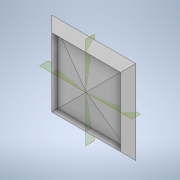
# Autodesk Inventor part: clear-square-inset
Saved by Autodesk Inventor 2021 (Build 250183000, 183)
## iProperties
Created: 2020-12-08
Part Number: clear-square-inset
Material: Generic
Document SubType Name: Modeling
Designer: Luke Kamols
Density: 1 g/cm^3
Appearance: Default
Author: Luke Kamols
Autodesk Inventor part; units mm, degrees
ref_plane "YZ Plane" through (0, 0, 0) normal (1, 0, 0) x (0, 1, 0)
ref_plane "XZ Plane" through (0, 0, 0) normal (0, 1, 0) x (-1, 0, 0)
ref_plane "XY Plane" through (0, 0, 0) normal (0, 0, 1) x (1, 0, 0)
sketch "Sketch1" plane through (0, 0, 0) normal (0, 0, 1) x (1, 0, 0)
  line L0 (0, 0) -> (44, 0)
  line L1 (44, 0) -> (44, 44)
  line L2 (44, 44) -> (0, 44)
  line L3 (0, 44) -> (0, 0)
  dimension "d0" = 44
  dimension "d1" = 44
  constraints: 8 end point, 2 parallel, 1 horizontal, 1 perpendicular
  measures "d0" distance of L2.end L1.end
  measures "d1" distance of L1.end L0.end
extrude "Extrusion1" add sketch "Sketch1" along normal blind 4
chamfer "Chamfer1" distance 4 angle 45 4 edges at (22, 44, 4) (44, 22, 4) (22, 0, 4) (0, 22, 4)
ref_plane "Work Plane1" through (0, 22, 22) normal (0, -1, 0) x (1, 0, 0)
sketch "Sketch5" plane through (0, 22, 22) normal (0, -1, 0) x (1, 0, 0)
  line L0 (40, -18) -> (4, -18) projected
  line L1 (4, -18) -> (0, -22) projected
  line L2 (0, -22) -> (44, -22) projected
  line L3 (40, -18) -> (44, -22) projected
  line L4 (4, -18) -> (4, -22)
  line L5 (40, -18) -> (40, -22)
  line L6 (40, -22) -> (40, -21)
  line L7 (40, -21) -> (22, -18)
  line L8 (4, -22) -> (4, -21)
  line L9 (22, -18) -> (4, -21)
  dimension "d25" = 1
  constraints: 12 end point, 4 point on line, 2 vertical, 1 midpoint
  measures "d25" distance of L5.end L6.end
extrude "Extrusion4" cut sketch "Sketch5" against normal mid plane 36 contours L5 L7 L0 | L9 L4 L0
ref_plane "Work Plane2" through (22, 0, 22) normal (-1, 0, 0) x (0, -1, 0)
sketch "Sketch6" plane through (22, 0, 22) normal (-1, 0, 0) x (0, -1, 0)
  line L0 (-4, -18) -> (-40, -18) projected
  line L1 (-4, -18) -> (-4, -21) projected
  line L2 (-40, -21) -> (-40, -18) projected
  line L3 (-40, -21) -> (-4, -21) projected
  line L4 (-4, -21) -> (-22, -18)
  line L5 (-40, -18) -> (-4, -18) projected
  line L6 (-4, -21) -> (-40, -21) projected
  line L7 (-40, -21) -> (-22, -18)
  point P0 (0, -22)
  constraints: 4 end point, 1 midpoint
extrude "Extrusion5" cut sketch "Sketch6" along normal mid plane 36 contours L1 L4 L0 | L7 L2 L0
body "Solid1"
